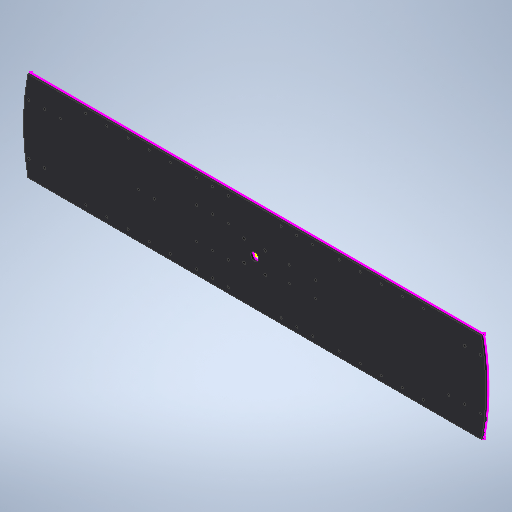
# Autodesk Inventor part: RotorV2
Saved by Autodesk Inventor 2025 (Build 290162000, 162)
## iProperties
Created: 2025-11-23
Part Number: RotorV2
Material: Generic
Document SubType Name: Modeling
Designer: ruven
Density: 1 g/cm^3
Appearance: Default
Author: ruven
Autodesk Inventor part; units mm, degrees
ref_plane "YZ Plane" through (0, 0, 0) normal (1, 0, 0) x (0, 1, 0)
ref_plane "XZ Plane" through (0, 0, 0) normal (0, 1, 0) x (-1, 0, 0)
ref_plane "XY Plane" through (0, 0, 0) normal (0, 0, 1) x (1, 0, 0)
sketch "Sketch1" plane through (0, 0, 0) normal (0, 1, 0) x (-1, 0, 0)
  line L0 (-438.1, 85) -> (438.1, 85)
  line L1 (438.1, 85) -> (438.1, -85)
  line L2 (438.1, -85) -> (-438.1, -85)
  line L3 (-438.1, -85) -> (-438.1, 85)
  line L4 (-438.1, 85) -> (438.1, -85) construction
  line L5 (438.1, 85) -> (-438.1, -85) construction
  point P0 (0, 0)
  dimension "d0" = 876.2
  dimension "d1" = 170
  constraints: 12 end point, 2 midpoint, 2 parallel, 1 horizontal, 1 perpendicular
  measures "d0" distance of L1.end L2.end
  measures "d1" distance between parallel lines of L0 L2
extrude "Extrusion1" add sketch "Sketch1" along normal blind 5
sketch "Sketch2" plane through (0, 5, 0) normal (0, 1, 0) x (1, 0, 0)
  line L0 (-421.2576, -120.3063) -> (-479.2742, -135.6981)
  line L1 (-479.2742, -135.6981) -> (-482.0374, 181.5112)
  line L2 (-482.0374, 181.5112) -> (-421.2576, 120.3063)
  line L3 (393.0571, -193.4883) -> (511.4336, -241.3123)
  line L4 (511.4336, -241.3123) -> (507.278, 235.7508)
  line L5 (507.278, 235.7508) -> (421.2576, 120.3063)
  arc A0 (393.0571, -193.4883) -> (421.2576, 120.3063) centre (0, 0) ccw
  arc A1 (-421.2576, 120.3063) -> (-421.2576, -120.3063) centre (0, 0) ccw
  constraints: 12 end point, 4 point on circle, 2 centre point, 1 coincident, 1 parallel
extrude "Extrusion2" cut sketch "Sketch2" against normal through all
sketch "Sketch3" plane through (0, 5, 0) normal (0, 1, 0) x (1, 0, 0)
  circle A0 centre (0, 0) radius 7.5
  dimension "d6" = 15
  constraints: 1 centre point, 1 coincident
  measures "d6" diameter of A0
extrude "Extrusion3" cut sketch "Sketch3" against normal through all
sketch "Sketch4" plane through (0, 5, 0) normal (0, 1, 0) x (1, 0, 0)
  point P0 (0, 0)
sketch "Sketch5" plane through (0, 5, 0) normal (0, 1, 0) x (1, 0, 0)
  line L0 (30, -30) -> (-30, -30) construction
  line L1 (-30, -30) -> (-30, 30) construction
  line L2 (-30, 30) -> (30, 30) construction
  line L3 (30, 30) -> (30, -30) construction
  circle A0 centre (0, 0) radius 7.5 projected
  line L4 (30, -30) -> (-30, 30) construction
  line L5 (-30, -30) -> (30, 30) construction
  circle A1 centre (-20, -20) radius 2.5
  circle A2 centre (-20, 20) radius 2.5
  circle A3 centre (20, 20) radius 2.5
  circle A4 centre (20, -20) radius 2.5
  dimension "d9" = 60
  dimension "d10" = 60
  dimension "d11" = 5
  dimension "d12" = 5
  dimension "d13" = 5
  dimension "d14" = 5
  dimension "d15" = 10
  dimension "d16" = 10
  dimension "d17" = 10
  dimension "d18" = 10
  constraints: 12 end point, 4 centre point, 4 point on line, 2 midpoint, 2 parallel, 1 horizontal, 1 perpendicular
  measures "d9" distance of L0.start L0.end
  measures "d10" distance of L0.end L1.end
  measures "d11" diameter of A1
  measures "d12" diameter of A2
  measures "d13" diameter of A3
  measures "d14" diameter of A4
  measures "d15" distance from line of L0 A1.centre
  measures "d16" distance from line of L2 A2.centre
  measures "d17" distance from line of L2 A3.centre
  measures "d18" distance from line of L3 A4.centre
extrude "Extrusion4" cut sketch "Sketch5" against normal through all contours A1 | A2 | A3 | A4
sketch "Sketch6" plane through (0, 5, 0) normal (0, 1, 0) x (1, 0, 0)
  circle A0 centre (-428.0999, -43.1) radius 2
  circle A1 centre (-428.0999, 53.1) radius 2.5
  line L0 (-377.1739, 38.1) -> (-433.9276, 38.1) construction
  line L1 (-433.9276, 38.1) -> (-433.9276, -38.1) construction
  line L2 (-433.9276, -38.1) -> (-377.1739, -38.1) construction
  line L3 (-377.1739, -38.1) -> (-377.1739, 38.1) construction
  line L4 (-377.1739, 38.1) -> (-433.9276, -38.1) construction
  line L5 (-433.9276, 38.1) -> (-377.1739, -38.1) construction
  line L6 (0, 0) -> (-428.0999, -43.1) construction
  line L7 (-429.7751, -85) -> (429.7751, -85) projected
  line L8 (-428.0999, -43.1) -> (-428.0999, 53.1) construction
  circle A2 centre (-398.0999, -43.1) radius 2
  circle A3 centre (-368.0999, -43.1) radius 2
  circle A4 centre (-398.0999, 53.1) radius 2.5
  line L9 (0, -85) -> (0, 85) construction
  line L10 (429.7751, 85) -> (-429.7751, 85) projected
  line L11 (377.1739, 38.1) -> (433.9276, 38.1) construction
  line L12 (438.1, 0) -> (328.0571, 0)
  circle A5 centre (428.0999, 43.1) radius 2
  circle A6 centre (398.0999, 43.1) radius 2
  circle A7 centre (368.0999, 43.1) radius 2
  circle A8 centre (398.0999, -53.1) radius 2.5
  circle A9 centre (428.0999, -53.1) radius 2.5
  point P0 (-405.5507, 0)
  dimension "d21" = 4
  dimension "d22" = 5
  dimension "d23" = 96.2
  dimension "d27" = 85
  dimension "d28" = 90
  dimension "d29" = 430.264
  dimension "d30" = 4
  dimension "d31" = 4
  dimension "d32" = 5
  dimension "d33" = 30
  dimension "d34" = 30
  dimension "d35" = 30
  dimension "d36" = 81.2
  dimension "d37" = 81.2
  dimension "d38" = 81.2
  dimension "d39" = 76.2
  dimension "d40" = 15
  constraints: 22 end point, 10 centre point, 4 midpoint, 2 horizontal, 2 parallel, 2 symmetric about line, 1 perpendicular
  measures "d21" diameter of A0
  measures "d22" diameter of A1
  measures "d23" distance of L8.end L6.end
  measures "d27" distance from line of L7 point (-405.551, 0)
  measures "d28" angle of L2 L8
  measures "d29" distance of L6.start L6.end
  measures "d30" diameter of A2
  measures "d31" diameter of A3
  measures "d32" diameter of A4
  measures "d33" distance of L6.end A2.centre
  measures "d34" distance of A3.centre A2.centre
  measures "d35" distance of L8.end A4.centre
  measures "d36" distance from line of L0 L6.end
  measures "d37" distance from line of L0 A2.centre
  measures "d38" distance from line of L0 A3.centre
  measures "d39" distance between parallel lines of L0 L2
  measures "d40" distance from line of L0 A4.centre
extrude "Extrusion5" cut sketch "Sketch6" against normal through all
sketch "Sketch7" plane through (0, 5, 0) normal (0, 1, 0) x (1, 0, 0)
  circle A0 centre (-110, -75) radius 2
  circle A1 centre (-80, -75) radius 2
  circle A2 centre (-50, -75) radius 2
  circle A3 centre (-110, 75) radius 2
  circle A4 centre (-80, 75) radius 2
  circle A5 centre (-50, 75) radius 2
  line L0 (-429.7751, -85) -> (429.7751, -85) projected
  line L1 (0, -85) -> (0, 85)
  line L2 (429.7751, 85) -> (-429.7751, 85) projected
  circle A6 centre (110, -75) radius 2
  circle A7 centre (80, -75) radius 2
  circle A8 centre (50, -75) radius 2
  circle A9 centre (110, 75) radius 2
  circle A10 centre (80, 75) radius 2
  circle A11 centre (50, 75) radius 2
  point P0 (0, 0)
  point P1 (0, 0)
  dimension "d43" = 4
  dimension "d44" = 4
  dimension "d45" = 4
  dimension "d46" = 4
  dimension "d47" = 4
  dimension "d48" = 4
  dimension "d49" = 30
  dimension "d56" = 30
  dimension "d58" = 50
  dimension "d126" = 10
  dimension "d127" = 10
  dimension "d128" = 10
  dimension "d129" = 30
  dimension "d130" = 30
  dimension "d131" = 50
  dimension "d132" = 10
  constraints: 12 centre point, 6 symmetric about line, 3 midpoint, 2 end point, 6 other
  measures "d43" diameter of A0
  measures "d44" diameter of A1
  measures "d45" diameter of A2
  measures "d46" diameter of A3
  measures "d47" diameter of A4
  measures "d48" diameter of A5
  measures "d49" distance of A1.centre A0.centre
  measures "d56" distance of A4.centre A3.centre
  measures "d58" horizontal distance of point (0, 0) A2.centre
  measures "d126" distance from line of L0 A0.centre
  measures "d127" distance from line of L0 A1.centre
  measures "d128" distance from line of L0 A2.centre
  measures "d129" distance of A1.centre A2.centre
  measures "d130" distance of A5.centre A4.centre
  measures "d131" horizontal distance of point (0, 0) A5.centre
  measures "d132" distance from line of L2 A5.centre
extrude "Extrusion6" cut sketch "Sketch7" against normal through all
sketch "Sketch8" plane through (0, 0, 0) normal (0, -1, 0) x (1, 0, 0)
  circle A0 centre (-160, 75) radius 2
  circle A1 centre (-200, 75) radius 2
  circle A2 centre (-240, 75) radius 2
  circle A3 centre (-280, 75) radius 2
  circle A4 centre (-320, 75) radius 2
  circle A5 centre (-110, 75) radius 2 projected
  line L0 (-429.7751, 85) -> (429.7751, 85) projected
  line L1 (-390.896, 0) -> (65.5505, 0)
  line L2 (0, 85) -> (0, -85)
  line L3 (429.7751, -85) -> (-429.7751, -85) projected
  circle A6 centre (-160, -75) radius 2
  circle A7 centre (-200, -75) radius 2
  circle A8 centre (-240, -75) radius 2
  circle A9 centre (-280, -75) radius 2
  circle A10 centre (-320, -75) radius 2
  circle A11 centre (160, 75) radius 2
  circle A12 centre (200, 75) radius 2
  circle A13 centre (240, 75) radius 2
  circle A14 centre (280, 75) radius 2
  circle A15 centre (320, 75) radius 2
  circle A16 centre (320, -75) radius 2
  circle A17 centre (280, -75) radius 2
  circle A18 centre (240, -75) radius 2
  circle A19 centre (200, -75) radius 2
  circle A20 centre (160, -75) radius 2
  point P0 (0, 0)
  dimension "d61" = 4
  dimension "d62" = 4
  dimension "d63" = 4
  dimension "d64" = 4
  dimension "d65" = 4
  dimension "d66" = 40
  dimension "d67" = 40
  dimension "d68" = 40
  dimension "d69" = 40
  dimension "d70" = 50
  dimension "d71" = 10
  dimension "d72" = 10
  dimension "d73" = 10
  dimension "d74" = 10
  dimension "d75" = 10
  constraints: 20 centre point, 15 symmetric about line, 4 end point, 2 midpoint, 1 horizontal, 15 other
  measures "d61" diameter of A0
  measures "d62" diameter of A1
  measures "d63" diameter of A2
  measures "d64" diameter of A3
  measures "d65" diameter of A4
  measures "d66" distance of A1.centre A0.centre
  measures "d67" distance of A2.centre A1.centre
  measures "d68" distance of A2.centre A3.centre
  measures "d69" distance of A3.centre A4.centre
  measures "d70" distance of A5.centre A0.centre
  measures "d71" distance from line of L0 A0.centre
  measures "d72" distance from line of L0 A1.centre
  measures "d73" distance from line of L0 A2.centre
  measures "d74" distance from line of L0 A3.centre
  measures "d75" distance from line of L0 A4.centre
extrude "Extrusion7" cut sketch "Sketch8" against normal through all contours A0 | A1 | A2 | A3 | A4 | A6 | A7 | A8 | A9 | A10 | A11 | A12 | A13 | A14 | A15 | A16 | A17 | A18 | A19 | A20
sketch "Sketch10" plane through (0, 0, 0) normal (0, -1, 0) x (1, 0, 0)
  circle A0 centre (428.0999, -43.1) radius 2 projected
  line L0 (428.0999, -43.1) -> (428.0999, -76.869)
  line L1 (429.7751, -85) -> (-429.7751, -85) projected
  circle A1 centre (-428.0999, 43.1) radius 2 projected
  line L2 (-428.0999, 43.1) -> (-428.0999, 76.869)
  line L3 (-428.0999, 76.869) -> (96.8155, 49.3593) construction
  line L4 (-429.7751, 85) -> (429.7751, 85) projected
  line L5 (80, 50.2406) -> (80, -58.6259) construction
  line L6 (80, -58.6259) -> (80, 4.1931) construction
  circle A2 centre (80, 4.1931) radius 2.5 construction
  line L7 (120.525, -15.8069) -> (60.525, -15.8069) construction
  line L8 (60.525, -15.8069) -> (60.525, 24.1931) construction
  line L9 (60.525, 24.1931) -> (120.525, 24.1931) construction
  line L10 (120.525, 24.1931) -> (120.525, -15.8069) construction
  line L11 (120.525, -15.8069) -> (60.525, 24.1931) construction
  line L12 (60.525, -15.8069) -> (120.525, 24.1931) construction
  circle A3 centre (65.525, 19.1931) radius 2
  circle A4 centre (65.525, -10.8069) radius 2
  circle A5 centre (115.525, -10.8069) radius 2
  circle A6 centre (115.525, 19.1931) radius 2
  line L13 (428.0999, -76.869) -> (80, -58.6259)
  point P0 (0, 0)
  point P1 (90.525, 4.1931)
  point P2 (80, -4.1926)
  dimension "d83" = 33.769
  dimension "d84" = 33.769
  dimension "d86" = 177
  dimension "d87" = 80
  dimension "d88" = 108.8665
  dimension "d91" = 5
  dimension "d92" = 60
  dimension "d93" = 40
  dimension "d95" = 19.475
  dimension "d96" = 4
  dimension "d97" = 4
  dimension "d98" = 4
  dimension "d99" = 4
  dimension "d100" = 5
  dimension "d101" = 5
  dimension "d102" = 5
  dimension "d103" = 5
  dimension "d104" = 5
  dimension "d105" = 5
  dimension "d106" = 5
  dimension "d107" = 5
  dimension "d110" = 177
  dimension "d133" = 20
  dimension "d135" = 62.819
  constraints: 24 end point, 5 centre point, 3 midpoint, 2 parallel, 2 perpendicular, 2 point on line, 2 vertical, 1 coincident, 1 horizontal
  measures "d83" distance of L0.start L0.end
  measures "d84" distance of L2.start L2.end
  measures "d86" angle of L4 L3
  measures "d87" distance from line of L5 point (0, 0)
  measures "d88" distance of L5.start L5.end
  measures "d91" diameter of A2
  measures "d92" distance of L8.end L9.end
  measures "d93" distance of L7.end L8.end
  measures "d95" distance from line of point (80, -4.193) L8
  measures "d96" diameter of A3
  measures "d97" diameter of A4
  measures "d98" diameter of A5
  measures "d99" diameter of A6
  measures "d100" distance from line of L9 A3.centre
  measures "d101" distance from line of L8 A3.centre
  measures "d102" distance from line of L8 A4.centre
  measures "d103" distance from line of L7 A4.centre
  measures "d104" distance from line of L10 A5.centre
  measures "d105" distance from line of L7 A5.centre
  measures "d106" distance from line of L10 A6.centre
  measures "d107" distance from line of L9 A6.centre
  measures "d110" angle of L1 L13
  measures "d133" distance from line of A2.centre L9
  measures "d135" distance of L5.end A2.centre
extrude "Extrusion8" cut sketch "Sketch10" against normal blind 10 contours A3 | A4 | A5 | A6
sketch "Sketch11" plane through (0, 0, 0) normal (0, -1, 0) x (1, 0, 0)
  circle A0 centre (-110, 30) radius 2
  circle A1 centre (-80, 30) radius 2
  circle A2 centre (-50, 30) radius 2
  circle A3 centre (-50, -30) radius 2
  circle A4 centre (-80, -30) radius 2
  circle A5 centre (-110, -30) radius 2
  point P0 (0, 0)
  dimension "d111" = 30
  dimension "d112" = 30
  dimension "d113" = 30
  dimension "d114" = 30
  dimension "d115" = 30
  dimension "d116" = 30
  dimension "d117" = 4
  dimension "d118" = 4
  dimension "d119" = 4
  dimension "d120" = 4
  dimension "d121" = 4
  dimension "d122" = 4
  dimension "d123" = 30
  constraints: 6 centre point
  measures "d111" vertical distance of point (0, 0) A2.centre
  measures "d112" vertical distance of point (0, 0) A1.centre
  measures "d113" vertical distance of point (0, 0) A0.centre
  measures "d114" vertical distance of point (0, 0) A5.centre
  measures "d115" vertical distance of point (0, 0) A4.centre
  measures "d116" vertical distance of point (0, 0) A3.centre
  measures "d117" diameter of A2
  measures "d118" diameter of A1
  measures "d119" diameter of A0
  measures "d120" diameter of A3
  measures "d121" diameter of A4
  measures "d122" diameter of A5
  measures "d123" distance of A1.centre A0.centre
extrude "Extrusion9" cut sketch "Sketch11" against normal through all
sketch "Sketch12" plane through (0, 0, 0) normal (0, -1, 0) x (1, 0, 0)
  circle A0 centre (-220, 0) radius 2
  circle A1 centre (-190, 0) radius 2
  circle A2 centre (0, 0) radius 7.5 projected
  dimension "d136" = 190
  dimension "d137" = 220
  dimension "d138" = 4
  dimension "d139" = 4
  constraints: 2 centre point
  measures "d136" distance of A2.centre A1.centre
  measures "d137" distance of A2.centre A0.centre
  measures "d138" diameter of A1
  measures "d139" diameter of A0
extrude "Extrusion10" cut sketch "Sketch12" against normal blind 10 contours A0 | A1
sketch "Sketch13" plane through (0, 5, 0) normal (0, 1, 0) x (1, 0, 0)
  circle A0 centre (-190, 0) radius 2 projected
  circle A1 centre (-220, 0) radius 2 projected
  circle A2 centre (-50, 30) radius 2 projected
  circle A3 centre (-110, -30) radius 2 projected
  circle A4 centre (-50, -30) radius 2 projected
  circle A5 centre (-80, -30) radius 2 projected
  circle A6 centre (-80, 30) radius 2 projected
  circle A7 centre (-110, 30) radius 2 projected
  circle A8 centre (65.525, -19.1931) radius 2 projected
  circle A9 centre (115.525, 10.8069) radius 2 projected
  circle A10 centre (65.525, 10.8069) radius 2 projected
  circle A11 centre (115.525, -19.1931) radius 2 projected
  circle A12 centre (-200, -75) radius 2 projected
  circle A13 centre (-320, 75) radius 2 projected
  circle A14 centre (200, -75) radius 2 projected
  circle A15 centre (160, -75) radius 2 projected
  circle A16 centre (280, 75) radius 2 projected
  circle A17 centre (280, -75) radius 2 projected
  circle A18 centre (240, 75) radius 2 projected
  circle A19 centre (-240, -75) radius 2 projected
  circle A20 centre (-240, 75) radius 2 projected
  circle A21 centre (-280, -75) radius 2 projected
  circle A22 centre (-160, 75) radius 2 projected
  circle A23 centre (-160, -75) radius 2 projected
  circle A24 centre (320, 75) radius 2 projected
  circle A25 centre (200, 75) radius 2 projected
  circle A26 centre (320, -75) radius 2 projected
  circle A27 centre (160, 75) radius 2 projected
  circle A28 centre (240, -75) radius 2 projected
  circle A29 centre (-320, -75) radius 2 projected
  circle A30 centre (-200, 75) radius 2 projected
  circle A31 centre (-280, 75) radius 2 projected
  circle A32 centre (80, 75) radius 2 projected
  circle A33 centre (-50, 75) radius 2 projected
  circle A34 centre (-80, -75) radius 2 projected
  circle A35 centre (-50, -75) radius 2 projected
  circle A36 centre (110, -75) radius 2 projected
  circle A37 centre (110, 75) radius 2 projected
  circle A38 centre (50, -75) radius 2 projected
  circle A39 centre (-110, 75) radius 2 projected
  circle A40 centre (-110, -75) radius 2 projected
  circle A41 centre (-80, 75) radius 2 projected
  circle A42 centre (50, 75) radius 2 projected
  circle A43 centre (80, -75) radius 2 projected
  circle A44 centre (398.0999, 43.1) radius 2 projected
  circle A45 centre (-368.0999, -43.1) radius 2 projected
  circle A46 centre (-428.0999, -43.1) radius 2 projected
  circle A47 centre (-398.0999, 53.1) radius 2.5 projected
  circle A48 centre (368.0999, 43.1) radius 2 projected
  circle A49 centre (428.0999, 43.1) radius 2 projected
  circle A50 centre (-398.0999, -43.1) radius 2 projected
  circle A51 centre (-428.0999, 53.1) radius 2.5 projected
  circle A52 centre (398.0999, -53.1) radius 2.5 projected
  circle A53 centre (428.0999, -53.1) radius 2.5 projected
  circle A54 centre (-20, 20) radius 2.5 projected
  circle A55 centre (-20, -20) radius 2.5 projected
  circle A56 centre (20, 20) radius 2.5 projected
  circle A57 centre (20, -20) radius 2.5 projected
  circle A58 centre (0, 0) radius 7.5 projected
  arc A59 (-429.7751, 85) -> (-429.7751, -85) centre (0, 0) ccw projected
  line L0 (-429.7751, -85) -> (429.7751, -85) projected
  arc A60 (429.7751, -85) -> (429.7751, 85) centre (0, 0) ccw projected
  line L1 (429.7751, 85) -> (-429.7751, 85) projected
  line L2 (429.7751, 85) -> (-429.7751, 85) projected
  circle A61 centre (-190, 0) radius 2 projected
  circle A62 centre (-220, 0) radius 2 projected
  circle A63 centre (-50, 30) radius 2 projected
  circle A64 centre (-110, -30) radius 2 projected
  circle A65 centre (-50, -30) radius 2 projected
  circle A66 centre (-80, -30) radius 2 projected
  circle A67 centre (-80, 30) radius 2 projected
  circle A68 centre (-110, 30) radius 2 projected
  circle A69 centre (65.525, -19.1931) radius 2 projected
  circle A70 centre (115.525, 10.8069) radius 2 projected
  circle A71 centre (65.525, 10.8069) radius 2 projected
  circle A72 centre (115.525, -19.1931) radius 2 projected
  circle A73 centre (-200, -75) radius 2 projected
  circle A74 centre (-320, 75) radius 2 projected
  circle A75 centre (200, -75) radius 2 projected
  circle A76 centre (160, -75) radius 2 projected
  circle A77 centre (280, 75) radius 2 projected
  circle A78 centre (280, -75) radius 2 projected
  circle A79 centre (240, 75) radius 2 projected
  circle A80 centre (-240, -75) radius 2 projected
  circle A81 centre (-240, 75) radius 2 projected
  circle A82 centre (-280, -75) radius 2 projected
  circle A83 centre (-160, 75) radius 2 projected
  circle A84 centre (-160, -75) radius 2 projected
  circle A85 centre (320, 75) radius 2 projected
  circle A86 centre (200, 75) radius 2 projected
  circle A87 centre (320, -75) radius 2 projected
  circle A88 centre (160, 75) radius 2 projected
  circle A89 centre (240, -75) radius 2 projected
  circle A90 centre (-320, -75) radius 2 projected
  circle A91 centre (-200, 75) radius 2 projected
  circle A92 centre (-280, 75) radius 2 projected
  circle A93 centre (80, 75) radius 2 projected
  circle A94 centre (-50, 75) radius 2 projected
  circle A95 centre (-80, -75) radius 2 projected
  circle A96 centre (-50, -75) radius 2 projected
  circle A97 centre (110, -75) radius 2 projected
  circle A98 centre (110, 75) radius 2 projected
  circle A99 centre (50, -75) radius 2 projected
  circle A100 centre (-110, 75) radius 2 projected
  circle A101 centre (-110, -75) radius 2 projected
  circle A102 centre (-80, 75) radius 2 projected
  circle A103 centre (50, 75) radius 2 projected
  circle A104 centre (80, -75) radius 2 projected
  circle A105 centre (398.0999, 43.1) radius 2 projected
  circle A106 centre (-368.0999, -43.1) radius 2 projected
  circle A107 centre (-428.0999, -43.1) radius 2 projected
  circle A108 centre (-398.0999, 53.1) radius 2.5 projected
  circle A109 centre (368.0999, 43.1) radius 2 projected
  circle A110 centre (428.0999, 43.1) radius 2 projected
  circle A111 centre (-398.0999, -43.1) radius 2 projected
  circle A112 centre (-428.0999, 53.1) radius 2.5 projected
  circle A113 centre (398.0999, -53.1) radius 2.5 projected
  circle A114 centre (428.0999, -53.1) radius 2.5 projected
  circle A115 centre (-20, 20) radius 2.5 projected
  circle A116 centre (-20, -20) radius 2.5 projected
  circle A117 centre (20, 20) radius 2.5 projected
  circle A118 centre (20, -20) radius 2.5 projected
  circle A119 centre (0, 0) radius 7.5 projected
  arc A120 (-429.7751, 85) -> (-429.7751, -85) centre (0, 0) ccw projected
  line L3 (-429.7751, -85) -> (429.7751, -85) projected
  arc A121 (429.7751, -85) -> (429.7751, 85) centre (0, 0) ccw projected
  line L4 (429.7751, 85) -> (-429.7751, 85) projected
body "Solid1"
